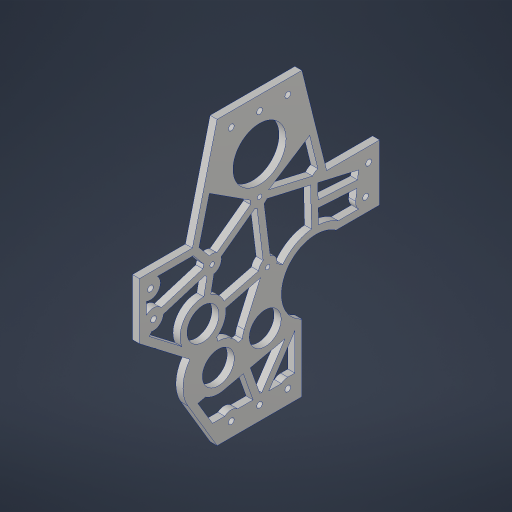
# Autodesk Inventor part: EL2-CGB-003
Saved by Autodesk Inventor 2023.4 (Build 274418000, 418)
## iProperties
Created: 2025-01-19
Part Number: EL2-CGB-003
Material: Aluminum 6061
Document SubType Name: Modeling
Designer: mavericks
Density: 2.7 g/cm^3
Appearance: Aluminum - Flat
Mass: 449.498 g
Surface Area: 622.856 cm^2
Volume: 166.481 cm^3
Author: mavericks
Autodesk Inventor part; units mm, degrees
ref_plane "YZ Plane" through (0, 0, 0) normal (1, 0, 0) x (0, 1, 0)
ref_plane "XZ Plane" through (0, 0, 0) normal (0, 1, 0) x (-1, 0, 0)
ref_plane "XY Plane" through (0, 0, 0) normal (0, 0, 1) x (1, 0, 0)
sketch "Sketch1" plane through (0, 0, 0) normal (1, 0, 0) x (0, 1, 0)
  line L0 (127, 107.95) -> (-127, 107.95) construction
  line L1 (-127, 107.95) -> (-127, 82.55) construction
  line L2 (-127, 82.55) -> (127, 82.55) construction
  line L3 (127, 82.55) -> (127, 107.95) construction
  line L4 (-44.45, 128.7526) -> (-69.85, 128.7526) construction
  line L5 (-69.85, 128.7526) -> (-69.85, 79.4258) construction
  line L6 (-69.85, 79.4258) -> (-44.45, 79.4258) construction
  line L7 (-44.45, 79.4258) -> (-44.45, 128.7526) construction
  line L8 (69.85, 128.7526) -> (44.45, 128.7526) construction
  line L9 (44.45, 128.7526) -> (44.45, 79.4258) construction
  line L10 (44.45, 79.4258) -> (69.85, 79.4258) construction
  line L11 (69.85, 79.4258) -> (69.85, 128.7526) construction
  line L12 (44.45, 104.0892) -> (-44.45, 104.0892) construction
  line L13 (0, 0) -> (-27.2932, 0) construction
  line L14 (127, -107.95) -> (-127, -107.95) construction
  line L15 (-127, -107.95) -> (-127, -82.55) construction
  line L16 (-127, -82.55) -> (127, -82.55) construction
  line L17 (127, -82.55) -> (127, -107.95) construction
  line L18 (-44.45, -128.7526) -> (-69.85, -128.7526) construction
  line L19 (-69.85, -128.7526) -> (-69.85, -79.4258) construction
  line L20 (-69.85, -79.4258) -> (-44.45, -79.4258) construction
  line L21 (-44.45, -79.4258) -> (-44.45, -128.7526) construction
  line L22 (69.85, -128.7526) -> (44.45, -128.7526) construction
  line L23 (44.45, -128.7526) -> (44.45, -79.4258) construction
  line L24 (44.45, -79.4258) -> (69.85, -79.4258) construction
  line L25 (69.85, -79.4258) -> (69.85, -128.7526) construction
  line L26 (44.45, -104.0892) -> (-44.45, -104.0892) construction
  line L27 (127, 82.55) -> (101.6, 82.55) construction
  line L28 (101.6, 82.55) -> (101.6, -82.55) construction
  line L29 (101.6, -82.55) -> (127, -82.55) construction
  line L30 (127, -82.55) -> (127, 82.55) construction
  line L31 (-127, 82.55) -> (-101.6, 82.55) construction
  line L32 (-101.6, 82.55) -> (-101.6, -82.55) construction
  line L33 (-101.6, -82.55) -> (-127, -82.55) construction
  line L34 (-127, -82.55) -> (-127, 82.55) construction
  point P0 (0, 82.55)
  point P1 (0, 104.0892)
  point P2 (0, -82.55)
  point P3 (0, -104.0892)
  dimension "d0" = 254
  dimension "d1" = 25.4
  dimension "d2" = 82.55
  dimension "d3" = 25.4
  dimension "d4" = 49.3268
  dimension "d6" = 88.9
  dimension "d7" = 3.1242
  dimension "d8" = 25.4
  dimension "d9" = 25.4
  constraints: 70 end point, 16 symmetric about line, 12 parallel, 7 horizontal, 5 perpendicular, 4 midpoint, 2 vertical alignment, 1 horizontal alignment, 1 point on line
  measures "d0" distance of L2.end L1.end
  measures "d1" distance of L1.end L0.end
  measures "d2" vertical distance of L13.start L2.end
  measures "d3" distance of L6.end L5.end
  measures "d4" distance of L5.end L4.end
  measures "d6" distance of L4.start L8.end
  measures "d7" distance from line of L2 L6.end
  measures "d8" distance between parallel lines of L28 L30
  measures "d9" distance between parallel lines of L34 L32
sketch "Sketch2" plane through (0, 0, 0) normal (1, 0, 0) x (0, 1, 0)
  line L0 (-127, 107.95) -> (-127, 82.55) construction
  line L1 (44.45, 104.0892) -> (-44.45, 104.0892) construction
  line L2 (-127, 82.55) -> (127, 82.55) construction
  line L3 (127, 107.95) -> (-127, 107.95) construction
  line L4 (44.45, 79.4258) -> (69.85, 79.4258) construction
  line L5 (127, 82.55) -> (127, 107.95) construction
  line L6 (-69.85, 79.4258) -> (-44.45, 79.4258) construction
  line L7 (-44.45, 79.4258) -> (-44.45, 128.7526) construction
  line L8 (-69.85, 128.7526) -> (-69.85, 79.4258) construction
  line L9 (-44.45, 128.7526) -> (-69.85, 128.7526) construction
  line L10 (101.6, 82.55) -> (101.6, -82.55) construction
  line L11 (127, -82.55) -> (127, 82.55) construction
  line L12 (-127, -82.55) -> (127, -82.55) construction
  line L13 (127, -107.95) -> (-127, -107.95) construction
  line L14 (44.45, -104.0892) -> (-44.45, -104.0892) construction
  line L15 (-127, 82.55) -> (-101.6, 82.55) construction
  line L16 (-101.6, 82.55) -> (-101.6, -82.55) construction
  line L17 (-127, -82.55) -> (-127, 82.55) construction
  line L18 (-69.85, -79.4258) -> (-44.45, -79.4258) construction
  line L19 (-101.6, -82.55) -> (-127, -82.55) construction
  line L20 (-44.45, -79.4258) -> (-44.45, -128.7526) construction
  line L21 (-44.45, -128.7526) -> (-69.85, -128.7526) construction
  line L22 (-69.85, -128.7526) -> (-69.85, -79.4258) construction
  line L23 (-127, -107.95) -> (-127, -82.55) construction
  line L24 (44.45, -79.4258) -> (69.85, -79.4258) construction
  line L25 (44.45, -128.7526) -> (44.45, -79.4258) construction
  line L26 (101.6, -82.55) -> (127, -82.55) construction
  line L27 (69.85, -128.7526) -> (44.45, -128.7526) construction
  line L28 (69.85, -79.4258) -> (69.85, -128.7526) construction
  line L29 (127, -82.55) -> (127, -107.95) construction
  line L30 (69.85, 128.7526) -> (44.45, 128.7526) construction
  line L31 (44.45, 128.7526) -> (44.45, 79.4258) construction
  line L32 (69.85, 79.4258) -> (69.85, 128.7526) construction
  line L33 (127, 82.55) -> (101.6, 82.55) construction
  circle A0 centre (-38.1, -50.8) radius 7.62 construction
  circle A1 centre (-57.15, -5.08) radius 41.91 construction
  circle A2 centre (-57.15, -5.08) radius 11.43 construction
  circle A3 centre (-66.675, 37.0363) radius 31.75 construction
  circle A4 centre (-66.675, 37.0363) radius 15.24 construction
  circle A5 centre (-25.7473, 50.8) radius 27.94 construction
  circle A6 centre (-38.1, -50.8) radius 31.115 construction
  circle A7 centre (-38.1, -50.8) radius 10.16 construction
  circle A8 centre (-57.15, -5.08) radius 14.2875
  circle A9 centre (-66.675, 37.0363) radius 14.2875
  circle A10 centre (-25.7473, 50.8) radius 14.2875
  circle A11 centre (-25.7473, 50.8) radius 20.6375 construction
  circle A12 centre (-66.675, 37.0363) radius 20.6375 construction
  circle A13 centre (-57.15, -5.08) radius 20.6375 construction
  circle A14 centre (-38.1, -50.8) radius 17.4625 construction
  circle A15 centre (-38.1, -50.8) radius 25.4 construction
  line L34 (-41.275, -131.9276) -> (-41.275, -76.2508) construction
  line L35 (-41.275, -76.2508) -> (-73.025, -76.2508) construction
  line L36 (-73.025, -76.2508) -> (-73.025, -131.9276) construction
  line L37 (-73.025, -131.9276) -> (-41.275, -131.9276) construction
  line L38 (-127, -38.1) -> (-127, 38.1)
  line L39 (-127, 38.1) -> (-41.275, 38.1) construction
  line L40 (-41.275, 38.1) -> (-41.275, 104.0892) construction
  circle A16 centre (-38.1, -50.8) radius 31.115
  circle A17 centre (80.9686, 0) radius 23.8125
  circle A18 centre (80.9686, 0) radius 33.3375 construction
  line L41 (37.9487, 60.325) -> (127, 38.1)
  line L42 (127, 38.1) -> (127, -38.1)
  line L43 (127, -38.1) -> (37.9487, -60.325)
  line L44 (37.9487, -60.325) -> (37.9487, -107.95)
  line L45 (37.9487, -107.95) -> (-12.7, -107.95)
  line L46 (37.9487, 60.325) -> (37.9487, 107.95)
  line L47 (37.9487, 107.95) -> (-12.7, 107.95)
  arc A19 (-23.3654, 68.8297) -> (-38.2397, 37.5831) centre (-25.7473, 50.8) ccw construction
  arc A20 (43.4827, -39.6598) -> (88.1161, 54.1018) centre (80.9686, 0) ccw construction
  line L48 (-12.7, 107.95) -> (-47.625, 62.4363)
  line L49 (-82.9044, 64.325) -> (-127, 38.1)
  arc A21 (-47.625, 62.4363) -> (-82.9044, 64.325) centre (-66.675, 37.0363) ccw
  line L50 (-66.5052, -38.1) -> (-127, -38.1)
  line L51 (-12.7, -68.7717) -> (-12.7, -107.95)
  line L52 (-23.3654, 68.8297) -> (88.1161, 54.1018) construction
  line L53 (-38.2397, 37.5831) -> (43.4827, -39.6598) construction
  point P0 (25.2487, 98.0186)
  point P1 (0, 95.25)
  point P2 (25.2487, -98.0186)
  point P3 (0, -95.25)
  point P4 (-25.4, -95.25)
  point P5 (-25.4, 95.25)
  point P6 (127, -95.25)
  point P7 (127, 95.25)
  point P8 (0, -82.55)
  point P9 (-114.3, 25.4)
  point P10 (-114.3, 0)
  point P11 (-114.3, -25.4)
  point P12 (-101.6, 0)
  point P13 (-114.3, 82.55)
  point P14 (-38.1, -25.4)
  point P15 (-38.1, -33.3375)
  point P16 (-60.097, -38.1)
  point P17 (-53.223, -42.0688)
  point P18 (-60.097, -63.5)
  point P19 (-53.223, -59.5312)
  point P20 (-38.1, -76.2)
  point P21 (-38.1, -68.2625)
  point P22 (-16.103, -63.5)
  point P23 (-22.977, -59.5313)
  point P24 (-16.103, -38.1)
  point P25 (-22.977, -42.0688)
  point P26 (44.45, 104.0892)
  point P27 (-41.275, -81.7526)
  point P28 (-127, 0)
  point P29 (-127, 0)
  point P30 (101.6, 0)
  point P31 (114.3, 25.4)
  point P32 (114.3, 0)
  point P33 (114.3, -25.4)
  point P34 (114.3, 82.55)
  point P35 (127, 0)
  dimension "d13" = 63.5
  dimension "d33" = 34.925
  dimension "d34" = 50.8
  dimension "d10" = 15.24
  dimension "d11" = 83.82
  dimension "d12" = 22.86
  dimension "d14" = 30.48
  dimension "d15" = 55.88
  dimension "d16" = 62.23
  dimension "d19" = 63.5
  dimension "d23" = 20.32
  dimension "d24" = 28.575
  dimension "d26" = 25.4
  dimension "d27" = 25.4
  dimension "d28" = 25.4
  dimension "d29" = 25.4
  dimension "d30" = 6.35
  dimension "d31" = 6.35
  dimension "d32" = 6.35
  dimension "d37" = 360
  dimension "d41" = 3.175
  dimension "d42" = 76.2
  dimension "d60" = 101.7513
  dimension "d63" = 31.75
  dimension "d64" = 44.45
  dimension "d66" = 34.925
  dimension "d67" = 31.75
  dimension "d68" = 47.625
  dimension "d70" = 9.525
  dimension "d71" = 47.625
  dimension "d73" = 118.1903
  dimension "d74" = 12.7
  dimension "d75" = 36.3728
  dimension "d76" = 109.1438
  dimension "d78" = 9.9314
  dimension "d79" = 9.9314
  dimension "d137" = 12.7
  dimension "d149" = 205.5979
  dimension "d151" = 45.7518
  dimension "d152" = 112.4501
  dimension "d153" = 6.35
  constraints: 41 end point, 19 centre point, 18 vertical alignment, 14 coincident, 11 horizontal alignment, 11 midpoint, 10 point on circle, 9 point on line, 6 tangent, 3 perpendicular, 2 collinear, 2 equal radius, 2 horizontal, 1 vertical, 25 other
  measures "d10" diameter of A0
  measures "d11" diameter of A1
  measures "d12" diameter of A2
  measures "d14" diameter of A4
  measures "d15" diameter of A5
  measures "d16" diameter of A6
  measures "d19" distance from line of L16 A0.centre
  measures "d23" diameter of A7
  measures "d24" diameter of A8
  measures "d26" distance of point (-25.4, 95.25) point (0, 95.25)
  measures "d27" distance of point (25.249, 98.019) point (0, 95.25)
  measures "d28" distance of point (-114.3, 0) point (-114.3, 25.4)
  measures "d29" distance of point (-114.3, 0) point (-114.3, -25.4)
  measures "d30" radial gap between concentric circles of A10 A11
  measures "d31" radial gap between concentric circles of A9 A12
  measures "d32" radial gap between concentric circles of A8 A13
  measures "d41" distance between parallel lines of L20 L34
  measures "d42" distance of L38.start L38.end
  measures "d60" distance from line of L5 point (25.249, 98.019)
  measures "d63" distance from line of L12 A0.centre
  measures "d64" distance from line of L16 A1.centre
  measures "d66" distance from line of L16 point (-66.675, 37.036)
  measures "d67" distance from line of L2 A5.centre
  measures "d68" diameter of A17
  measures "d70" radial gap between concentric circles of A17 A18
  measures "d71" distance of L41.start L46.end
  measures "d73" distance of A17.centre A5.centre
  measures "d74" horizontal distance of point (25.249, 98.019) L46.end
  measures "d75" diameter of A19
  measures "d76" diameter of A20
  measures "d78" distance from line of point (25.249, 98.019) L3
  measures "d79" distance from line of L13 point (25.249, -98.019)
  measures "d137" distance from line of L51 point (0, -95.25)
  measures "d152" distance of L52.start L52.end
  measures "d153" distance from line of L40 L48.end
extrude "Extrusion1" add sketch "Sketch2" along normal blind 6.35 contours L38 L49 A21 L48 L47 L46 L41 L42 L43 L44 L45 L51 A16 L50
hole "Mount Holes" at (0, -101.6, 82.55) at (0, -127, 107.95) at (0, -69.85, 79.4258) at (0, -44.45, -79.4258) at (0, 44.45, -79.4258) at (0, 69.85, -79.4258) at (0, 44.45, -128.7526) at (0, 44.45, 128.7526) at (0, 25.2487, 98.0186) at (0, 0, 95.25) at (0, 25.2487, -98.0186) at (0, 0, -95.25) at (0, -25.4, -95.25) at (0, -25.4, 95.25) at (0, -114.3, 25.4) at (0, -114.3, 0) at (0, -114.3, -25.4) at (0, 114.3, 25.4) at (0, 114.3, 0) at (0, 114.3, -25.4) direction (1, 0, 0) diameter 5.1054 end through all clearance for "Flat Head Machine Screw (82)" size "#10" standard "Ansi Unified Screw Threads"
sketch "Sketch7" plane through (6.35, 0, 0) normal (1, 0, 0) x (0, 0, -1)
  circle A0 centre (0, 114.3) radius 2.5527 construction
  circle A1 centre (25.4, -114.3) radius 2.5527 construction
  circle A2 centre (-25.4, -114.3) radius 2.5527 construction
  circle A3 centre (98.0186, 25.2487) radius 2.5527 construction
  circle A4 centre (-98.0186, 25.2487) radius 2.5527 construction
  circle A5 centre (-95.25, 0) radius 2.5527 construction
  circle A6 centre (95.25, 0) radius 2.5527 construction
  circle A7 centre (0, -114.3) radius 2.5527 construction
  circle A8 centre (-25.4, 114.3) radius 2.5527 construction
  circle A9 centre (25.4, 114.3) radius 2.5527 construction
  circle A10 centre (5.08, -57.15) radius 14.2875 construction
  circle A11 centre (-37.0363, -66.675) radius 14.2875 construction
  circle A12 centre (-50.8, -25.7473) radius 14.2875 construction
  circle A13 centre (0, 80.9686) radius 23.8125 construction
  line L0 (38.1, -127) -> (-38.1, -127) construction
  line L1 (-38.1, -127) -> (-64.325, -82.9044) construction
  arc A14 (-62.4363, -47.625) -> (-64.325, -82.9044) centre (-37.0363, -66.675) ccw construction
  line L2 (-62.4363, -47.625) -> (-93.0211, -24.1557) construction
  arc A15 (-93.0211, -24.1557) -> (-94.6249, -22.925) centre (-95.25, -25.4) ccw construction
  line L3 (-94.6249, -22.925) -> (-107.95, -12.7) construction
  line L4 (-107.95, -12.7) -> (-107.95, 37.9487) construction
  line L5 (-107.95, 37.9487) -> (-60.325, 37.9487) construction
  line L6 (-60.325, 37.9487) -> (-38.1, 127) construction
  line L7 (-38.1, 127) -> (38.1, 127) construction
  line L8 (38.1, 127) -> (60.325, 37.9487) construction
  line L9 (60.325, 37.9487) -> (107.95, 37.9487) construction
  line L10 (107.95, 37.9487) -> (107.95, -12.7) construction
  line L11 (107.95, -12.7) -> (68.7717, -12.7) construction
  arc A16 (68.7717, -12.7) -> (38.1, -66.5052) centre (50.8, -38.1) ccw construction
  line L12 (38.1, -66.5052) -> (38.1, -127) construction
  circle A17 centre (0, 80.9686) radius 54.5719 construction
  circle A18 centre (-50.8, -25.7473) radius 18.1864 construction
  line L13 (-54.1018, 88.1161) -> (-68.8297, -23.3654) construction
  line L14 (-37.5831, -38.2397) -> (39.6598, 43.4827) construction
  circle A19 centre (5.08, -2.5527) radius 20.6375 construction
  line L15 (-4.4521, -30.1851) -> (53.1372, 30.744) construction
  circle A20 centre (-4.4521, -30.1851) radius 4.7625 construction
  circle A21 centre (53.1372, 30.744) radius 4.7625 construction
  point P0 (0, 0)
  dimension "d154" = 109.1438
  dimension "d155" = 36.3728
  dimension "d194" = 41.275
  dimension "d197" = 9.525
  dimension "d198" = 9.525
  constraints: 6 end point, 5 centre point, 4 coincident, 4 point on circle, 4 tangent, 1 parallel
  measures "d154" diameter of A17
  measures "d155" diameter of A18
  measures "d194" diameter of A19
  measures "d197" diameter of A20
  measures "d198" diameter of A21
hole "Hole4" [suppressed]
sketch "Sketch8" plane through (6.35, 0, 0) normal (1, 0, 0) x (0, 0, -1)
  circle A0 centre (0, 114.3) radius 2.5527 construction
  line L0 (0, 47.6504) -> (0, 114.3) construction
  point P0 (0, 0)
  dimension "d183" = 66.6496
  constraints: 2 end point, 1 vertical
  measures "d183" distance of L0.start L0.end
hole "Hole5" at (6.35, 47.6504, 0) direction (-1, 0, 0) diameter 3.9624 end through all thread size "10-32 UNF" class "2B" standard "ANSI Unified Screw Threads"
sketch "Sketch9" plane through (0, 0, 0) normal (-1, 0, 0) x (0, 0, 1)
  circle A0 centre (0, 47.6504) radius 1.9812 construction
  circle A1 centre (0, 114.3) radius 2.5527 construction
  circle A2 centre (-25.4, -114.3) radius 2.5527 construction
  circle A3 centre (25.4, -114.3) radius 2.5527 construction
  circle A4 centre (-98.0186, 25.2487) radius 2.5527 construction
  circle A5 centre (98.0186, 25.2487) radius 2.5527 construction
  circle A6 centre (95.25, 0) radius 2.5527 construction
  circle A7 centre (-95.25, 0) radius 2.5527 construction
  circle A8 centre (0, -114.3) radius 2.5527 construction
  circle A9 centre (25.4, 114.3) radius 2.5527 construction
  circle A10 centre (-25.4, 114.3) radius 2.5527 construction
  circle A11 centre (-5.08, -57.15) radius 14.2875 construction
  circle A12 centre (37.0363, -66.675) radius 14.2875 construction
  circle A13 centre (50.8, -25.7473) radius 14.2875 construction
  circle A14 centre (0, 80.9686) radius 23.8125 construction
  line L0 (38.1, -127) -> (-38.1, -127) construction
  line L1 (-38.1, -127) -> (-38.1, -66.5052) construction
  arc A15 (-38.1, -66.5052) -> (-68.7717, -12.7) centre (-50.8, -38.1) ccw construction
  line L2 (-68.7717, -12.7) -> (-107.95, -12.7) construction
  line L3 (-107.95, -12.7) -> (-107.95, 37.9487) construction
  line L4 (-107.95, 37.9487) -> (-60.325, 37.9487) construction
  line L5 (-60.325, 37.9487) -> (-38.1, 127) construction
  line L6 (-38.1, 127) -> (38.1, 127) construction
  line L7 (38.1, 127) -> (60.325, 37.9487) construction
  line L8 (60.325, 37.9487) -> (107.95, 37.9487) construction
  line L9 (107.95, 37.9487) -> (107.95, -12.7) construction
  line L10 (107.95, -12.7) -> (94.6249, -22.925) construction
  arc A16 (94.6249, -22.925) -> (93.0211, -24.1557) centre (95.25, -25.4) ccw construction
  line L11 (93.0211, -24.1557) -> (62.4363, -47.625) construction
  arc A17 (64.325, -82.9044) -> (62.4363, -47.625) centre (37.0363, -66.675) ccw construction
  line L12 (64.325, -82.9044) -> (38.1, -127) construction
  circle A18 centre (50.8, -25.7473) radius 14.2875 construction
  circle A19 centre (50.8, -25.7473) radius 18.1864 construction
  circle A20 centre (0, 80.9686) radius 54.5719 construction
  line L13 (54.1018, 88.1161) -> (68.8297, -23.3654) construction
  line L14 (-39.6598, 43.4827) -> (37.5831, -38.2397) construction
  circle A21 centre (17.6097, 2.7489) radius 13.6398 construction
  line L15 (-7.4011, -10.7665) -> (42.6205, 16.2642) construction
  line L16 (0, 80.9686) -> (50.8, -25.7473) construction
  line L17 (23.4558, 31.6947) -> (42.9832, -9.3265) construction
  point P0 (0, 0)
  point P1 (33.2195, 11.1841)
  dimension "d199" = 28.575
  dimension "d201" = 36.3728
  dimension "d202" = 109.1438
  dimension "d204" = 50.8
  dimension "d205" = 106.716
  dimension "d206" = 27.2796
  dimension "d207" = 56.8579
  dimension "d208" = 75
  constraints: 10 end point, 6 point on circle, 5 coincident, 5 tangent, 3 centre point, 3 point on line, 2 midpoint
  measures "d199" diameter of A13
  measures "d201" diameter of A19
  measures "d202" diameter of A20
  measures "d204" horizontal distance of A13.centre L16.start
  measures "d205" vertical distance of A13.centre A14.centre
  measures "d206" diameter of A21
  measures "d207" distance of L15.start L15.end
  measures "d208" angle of L14 L15
hole "Hole6" at (0, 16.2642, 42.6205) at (0, -10.7665, -7.4011) at (0, 16.2642, 42.6205) direction (1, 0, 0) diameter 3.9624 end through all thread size "10-32 UNF" class "2B" standard "ANSI Unified Screw Threads"
sketch "Sketch10" plane through (6.35, 0, 0) normal (1, 0, 0) x (0, 0, -1)
  circle A0 centre (7.4011, -10.7665) radius 1.9812 construction
  circle A1 centre (-42.6205, 16.2642) radius 1.9812 construction
  circle A2 centre (0, 47.6504) radius 1.9812 construction
  circle A3 centre (0, 114.3) radius 2.5527 construction
  circle A4 centre (25.4, -114.3) radius 2.5527 construction
  circle A5 centre (-25.4, -114.3) radius 2.5527 construction
  circle A6 centre (98.0186, 25.2487) radius 2.5527 construction
  circle A7 centre (-98.0186, 25.2487) radius 2.5527 construction
  circle A8 centre (-95.25, 0) radius 2.5527 construction
  circle A9 centre (95.25, 0) radius 2.5527 construction
  circle A10 centre (0, -114.3) radius 2.5527 construction
  circle A11 centre (-25.4, 114.3) radius 2.5527 construction
  circle A12 centre (25.4, 114.3) radius 2.5527 construction
  circle A13 centre (5.08, -57.15) radius 14.2875 construction
  circle A14 centre (-37.0363, -66.675) radius 14.2875 construction
  circle A15 centre (-50.8, -25.7473) radius 14.2875 construction
  circle A16 centre (0, 80.9686) radius 23.8125 construction
  line L0 (38.1, -127) -> (-38.1, -127) construction
  line L1 (-38.1, -127) -> (-64.325, -82.9044) construction
  arc A17 (-62.4363, -47.625) -> (-64.325, -82.9044) centre (-37.0363, -66.675) ccw construction
  line L2 (-62.4363, -47.625) -> (-93.0211, -24.1557) construction
  arc A18 (-93.0211, -24.1557) -> (-94.6249, -22.925) centre (-95.25, -25.4) ccw construction
  line L3 (-94.6249, -22.925) -> (-107.95, -12.7) construction
  line L4 (-107.95, -12.7) -> (-107.95, 37.9487) construction
  line L5 (-107.95, 37.9487) -> (-60.325, 37.9487) construction
  line L6 (-60.325, 37.9487) -> (-38.1, 127) construction
  line L7 (-38.1, 127) -> (38.1, 127) construction
  line L8 (38.1, 127) -> (60.325, 37.9487) construction
  line L9 (60.325, 37.9487) -> (107.95, 37.9487) construction
  line L10 (107.95, 37.9487) -> (107.95, -12.7) construction
  line L11 (107.95, -12.7) -> (68.7717, -12.7) construction
  arc A19 (68.7717, -12.7) -> (38.1, -66.5052) centre (50.8, -38.1) ccw construction
  line L12 (38.1, -66.5052) -> (38.1, -127) construction
  line L13 (-33.14, 120.65) -> (-55.365, 31.5987) construction
  line L14 (-55.365, 31.5987) -> (-101.6, 31.5987) construction
  line L15 (-101.6, 31.5987) -> (-101.6, -9.5686) construction
  line L16 (-101.6, -9.5686) -> (-91.4775, -17.3361) construction
  arc A20 (-88.4371, -19.6692) -> (-91.4775, -17.3361) centre (-95.25, -25.4) ccw construction
  line L17 (-88.4371, -19.6692) -> (-52.9641, -46.8895) construction
  arc A21 (-52.9641, -46.8895) -> (-58.8673, -79.6585) centre (-37.0363, -66.675) ccw construction
  line L18 (-58.8673, -79.6585) -> (-34.4884, -120.65) construction
  line L19 (-34.4884, -120.65) -> (31.75, -120.65) construction
  line L20 (31.75, -120.65) -> (31.75, -70.3602) construction
  arc A22 (70.6888, -6.35) -> (31.75, -70.3602) centre (50.8, -38.1) ccw construction
  line L21 (70.6888, -6.35) -> (101.6, -6.35) construction
  line L22 (101.6, -6.35) -> (101.6, 31.5987) construction
  line L23 (101.6, 31.5987) -> (55.365, 31.5987) construction
  line L24 (55.365, 31.5987) -> (33.14, 120.65) construction
  line L25 (33.14, 120.65) -> (-33.14, 120.65) construction
  circle A23 centre (0, 47.6504) radius 1.9812 construction
  circle A24 centre (0, 47.6504) radius 8.3312 construction
  circle A25 centre (98.0186, 25.2487) radius 8.9027 construction
  circle A26 centre (95.25, 0) radius 8.9027 construction
  circle A27 centre (7.4011, -10.7665) radius 8.3312 construction
  circle A28 centre (-42.6205, 16.2642) radius 8.3312 construction
  circle A29 centre (-50.8, -25.7473) radius 20.6375 construction
  circle A30 centre (-98.0186, 25.2487) radius 8.9027 construction
  circle A31 centre (-95.25, 0) radius 8.9027 construction
  circle A32 centre (5.08, -57.15) radius 20.6375 construction
  circle A33 centre (-37.0363, -66.675) radius 20.6375 construction
  circle A34 centre (25.4, -114.3) radius 8.9027 construction
  circle A35 centre (0, -114.3) radius 8.9027 construction
  circle A36 centre (-25.4, -114.3) radius 8.9027 construction
  line L26 (-32.484, -86.8041) -> (9.6324, -77.2791) construction
  circle A37 centre (0, -114.3) radius 2.5527 construction
  line L27 (0, -114.3) -> (-11.4258, -82.0416) construction
  circle A38 centre (7.4011, -10.7665) radius 1.9812 construction
  line L28 (-50.8, -25.7473) -> (7.4011, -10.7665) construction
  line L29 (7.4011, -10.7665) -> (50.8, -38.1) construction
  line L30 (-36.518, -25.3497) -> (6.8672, -14.1824) construction
  line L31 (6.8672, -14.1824) -> (75.2988, -57.2821) construction
  line L32 (-38.1009, -19.2001) -> (7.9351, -7.3505) construction
  line L33 (7.9351, -7.3505) -> (78.6829, -51.909) construction
  arc A39 (68.7717, -12.7) -> (38.1, -66.5052) centre (50.8, -38.1) ccw construction
  circle A40 centre (-50.8, -25.7473) radius 14.2875 construction
  line L34 (7.4011, -10.7665) -> (0, 47.6504) construction
  line L35 (0, 47.6504) -> (98.0186, 25.2487) construction
  line L36 (0, 47.6504) -> (-42.6205, 16.2642) construction
  line L37 (-42.6205, 16.2642) -> (-50.8, -25.7473) construction
  circle A41 centre (-42.6205, 16.2642) radius 1.9812 construction
  line L38 (-42.6205, 16.2642) -> (-55.365, 31.5987) construction
  circle A42 centre (-95.25, 0) radius 2.5527 construction
  line L39 (-95.25, 0) -> (-42.6205, 16.2642) construction
  line L40 (49.0093, 36.4495) -> (50.8, -38.1) construction
  line L41 (45.8945, 33.9045) -> (46.8826, -7.2326) construction
  line L42 (52.2814, 32.4448) -> (54.7174, -68.9674) construction
  line L43 (105.4194, 20.3004) -> (0.7111, 44.231) construction
  line L44 (0.7111, 44.231) -> (-39.7407, 14.4419) construction
  line L45 (-39.7407, 14.4419) -> (-50.3457, -40.0276) construction
  line L46 (-104.1339, 0.5777) -> (-48.1027, 17.8932) construction
  line L47 (-48.1027, 17.8932) -> (-59.4934, 31.5987) construction
  line L48 (-2.1817, 39.6099) -> (3.2832, -3.5241) construction
  line L49 (4.118, 40.4081) -> (9.5828, -2.726) construction
  line L50 (-13.8121, -48.8437) -> (0.7332, -15.7613) construction
  line L51 (-38.5221, -42.3353) -> (-37.2767, -46.0389) construction
  line L52 (-19.2845, -56.1499) -> (-15.4733, -55.288) construction
  line L53 (-37.0363, -66.675) -> (5.08, -57.15) construction
  line L54 (-50.8, -25.7473) -> (-37.0363, -66.675) construction
  line L55 (-5.7697, -107.52) -> (-14.5443, -82.7469) construction
  line L56 (5.7697, -121.08) -> (-8.3073, -81.3364) construction
  line L57 (-42.2972, -107.52) -> (31.75, -107.52) construction
  line L58 (-48.4099, -83.8956) -> (-55.4063, -85.4779) construction
  line L59 (45.8945, 33.9045) -> (46.7295, -0.8568)
  line L60 (4.118, 40.4081) -> (9.5828, -2.726)
  arc A43 (15.6107, -12.1848) -> (9.5828, -2.726) centre (7.4011, -10.7665) ccw
  line L61 (15.6107, -12.1848) -> (20.9047, -15.5191)
  arc A44 (46.7295, -0.8568) -> (20.9047, -15.5191) centre (50.8, -38.1) ccw
  line L62 (45.8945, 33.9045) -> (6.8015, 42.8391)
  arc A45 (4.118, 40.4081) -> (6.8015, 42.8391) centre (0, 47.6504) ccw
  line L63 (-4.3195, 40.5264) -> (-34.5356, 18.275)
  line L64 (-40.976, 8.0969) -> (-43.7865, -6.3381)
  line L65 (-31.8433, -17.5894) -> (-0.8496, -9.6117)
  line L66 (3.2832, -3.5241) -> (-2.1817, 39.6099)
  arc A46 (-4.3195, 40.5264) -> (-2.1817, 39.6099) centre (0, 47.6504) ccw
  arc A47 (-40.976, 8.0969) -> (-34.5356, 18.275) centre (-42.6205, 16.2642) ccw
  arc A48 (-31.8433, -17.5894) -> (-43.7865, -6.3381) centre (-50.8, -25.7473) ccw
  arc A49 (3.2832, -3.5241) -> (-0.8496, -9.6117) centre (7.4011, -10.7665) ccw
  line L67 (-86.3661, -0.5777) -> (-49.0421, 10.9565) construction
  line L68 (-50.0194, -5.1246) -> (-47.209, 9.3104) construction
  line L69 (-86.3661, -0.5777) -> (-49.0421, 10.9565)
  line L70 (-47.209, 9.3104) -> (-50.0194, -5.1246)
  line L71 (-99.0811, -11.5014) -> (-69.6924, -34.0529)
  line L72 (-96.9598, -8.737) -> (-99.0811, -11.5014) construction
  circle A50 centre (0, 80.9686) radius 30.1625 construction
  circle A51 centre (0, 47.6504) radius 1.9812 construction
  line L73 (0, 47.6504) -> (-44.2525, 76.1243) construction
  line L74 (0, 47.6504) -> (44.2525, 76.1243) construction
  line L75 (45.0644, 72.8713) -> (0, 43.8749) construction
  line L76 (0, 43.8749) -> (-45.0644, 72.8713) construction
  line L77 (-99.0811, -11.5014) -> (-96.9598, -8.737)
  arc A52 (-50.0194, -5.1246) -> (-69.6924, -34.0529) centre (-50.8, -25.7473) ccw
  arc A53 (-49.0421, 10.9565) -> (-47.209, 9.3104) centre (-42.6205, 16.2642) ccw
  arc A54 (-96.9598, -8.737) -> (-86.3661, -0.5777) centre (-95.25, 0) ccw
  line L78 (53.0777, -0.7043) -> (52.2814, 32.4448) construction
  line L79 (52.6795, 15.8703) -> (87.7846, 13.5947) construction
  line L80 (86.4003, 0.9704) -> (89.1689, 26.2191) construction
  line L81 (52.603, 19.0569) -> (88.1311, 16.7539) construction
  line L82 (52.7561, 12.6836) -> (87.4382, 10.4355) construction
  line L83 (87.4382, 10.4355) -> (52.7561, 12.6836)
  line L84 (52.7561, 12.6836) -> (53.0777, -0.7043)
  line L85 (87.4382, 10.4355) -> (86.4003, 0.9704)
  line L86 (89.0102, -6.35) -> (70.6888, -6.35)
  arc A55 (70.6888, -6.35) -> (53.0777, -0.7043) centre (50.8, -38.1) ccw
  circle A56 centre (95.25, 0) radius 2.5527 construction
  arc A57 (86.4003, 0.9704) -> (89.0102, -6.35) centre (95.25, 0) ccw
  line L87 (52.2814, 32.4448) -> (88.9331, 24.0682)
  line L88 (88.9331, 24.0682) -> (88.1311, 16.7539)
  line L89 (88.1311, 16.7539) -> (52.603, 19.0569)
  line L90 (52.603, 19.0569) -> (52.2814, 32.4448)
  line L91 (-38.301, 23.3881) -> (-8.0849, 45.6396) construction
  line L92 (8.2163, 49.0295) -> (53.6036, 38.6564) construction
  line L93 (-54.4116, 35.4188) -> (-45.1019, 24.2173) construction
  circle A58 centre (54.4656, 35.2025) radius 8.3312 construction
  line L94 (45.0644, 72.8713) -> (8.1955, 49.1482)
  line L95 (8.2163, 49.0295) -> (47.6641, 40.0138)
  line L96 (45.0644, 72.8713) -> (52.4482, 43.2858)
  arc A59 (52.4482, 43.2858) -> (47.6641, 40.0138) centre (54.4656, 35.2025) ccw
  arc A60 (8.2163, 49.0295) -> (8.1955, 49.1482) centre (0, 47.6504) ccw
  line L97 (-45.0644, 72.8713) -> (-54.4116, 35.4188)
  line L98 (-54.4116, 35.4188) -> (-45.1019, 24.2173)
  line L99 (-45.0644, 72.8713) -> (-8.1955, 49.1482)
  line L100 (-38.301, 23.3881) -> (-8.0849, 45.6396)
  arc A61 (-8.1955, 49.1482) -> (-8.0849, 45.6396) centre (0, 47.6504) ccw
  arc A62 (-38.301, 23.3881) -> (-45.1019, 24.2173) centre (-42.6205, 16.2642) ccw
  line L101 (-91.7788, 31.5987) -> (-59.4934, 31.5987)
  line L102 (-59.4934, 31.5987) -> (-49.9855, 20.1585)
  line L103 (-50.917, 17.0235) -> (-88.2409, 5.4892)
  line L104 (-101.6, 17.0981) -> (-101.6, 6.2398)
  arc A63 (-88.2409, 5.4892) -> (-101.6, 6.2398) centre (-95.25, 0) ccw
  arc A64 (-101.6, 17.0981) -> (-91.7788, 31.5987) centre (-98.0186, 25.2487) ccw
  arc A65 (-49.9855, 20.1585) -> (-50.917, 17.0235) centre (-42.6205, 16.2642) ccw
  line L105 (-30.2605, -23.739) -> (0.7332, -15.7613)
  line L106 (0.7332, -15.7613) -> (-13.8121, -48.8437)
  line L107 (-19.2845, -56.1499) -> (-15.4733, -55.288)
  line L108 (-38.5221, -42.3353) -> (-37.2767, -46.0389)
  circle A66 centre (-50.8, -25.7473) radius 14.2875 construction
  arc A67 (-38.5221, -42.3353) -> (-30.2605, -23.739) centre (-50.8, -25.7473) ccw
  arc A68 (-19.2845, -56.1499) -> (-37.2767, -46.0389) centre (-37.0363, -66.675) ccw
  circle A69 centre (5.08, -57.15) radius 14.2875 construction
  arc A70 (-13.8121, -48.8437) -> (-15.4733, -55.288) centre (5.08, -57.15) ccw
  line L109 (0, -114.3) -> (50.8, -38.1) construction
  line L110 (7.2554, -109.1408) -> (31.75, -72.3988) construction
  line L111 (1.9718, -105.6184) -> (27.4512, -67.3995) construction
  line L112 (-14.5443, -82.7469) -> (-5.7697, -107.52)
  line L113 (-5.7697, -107.52) -> (-19.6303, -107.52)
  line L114 (-14.5443, -82.7469) -> (-32.484, -86.8041)
  line L115 (-55.4063, -85.4779) -> (-48.4099, -83.8956)
  line L116 (-55.4063, -85.4779) -> (-42.2972, -107.52)
  line L117 (-42.2972, -107.52) -> (-31.1697, -107.52)
  arc A71 (-48.4099, -83.8956) -> (-32.484, -86.8041) centre (-37.0363, -66.675) ccw
  arc A72 (-19.6303, -107.52) -> (-31.1697, -107.52) centre (-25.4, -114.3) ccw
  line L118 (9.6324, -77.2791) -> (27.3522, -73.2716) construction
  line L119 (-8.3073, -81.3364) -> (22.8589, -74.2878)
  line L120 (22.8589, -74.2878) -> (1.9718, -105.6184)
  arc A73 (1.9718, -105.6184) -> (0.2159, -105.3999) centre (0, -114.3) ccw
  line L121 (-8.3073, -81.3364) -> (0.2159, -105.3999)
  line L122 (31.75, -72.3988) -> (8.3359, -107.52)
  line L123 (31.75, -72.3988) -> (31.75, -105.3973)
  line L124 (25.4, -105.3973) -> (31.75, -105.3973) construction
  line L125 (31.75, -105.3973) -> (25.4, -105.3973)
  circle A74 centre (25.4, -114.3) radius 2.5527 construction
  arc A75 (25.4, -105.3973) -> (19.6303, -107.52) centre (25.4, -114.3) ccw
  line L126 (19.6303, -107.52) -> (8.3359, -107.52)
  point P0 (0, 0)
  dimension "d258" = 16.6624
  dimension "d216" = 6.35
  dimension "d218" = 6.35
  dimension "d219" = 6.35
  dimension "d220" = 6.35
  dimension "d221" = 6.35
  dimension "d222" = 6.35
  dimension "d223" = 6.35
  dimension "d224" = 6.35
  dimension "d225" = 6.35
  dimension "d226" = 6.35
  dimension "d227" = 6.35
  dimension "d228" = 6.35
  dimension "d229" = 6.35
  dimension "d230" = 6.35
  dimension "d231" = 3.175
  dimension "d232" = 3.175
  dimension "d233" = 3.175
  dimension "d234" = 3.175
  dimension "d235" = 3.175
  dimension "d236" = 3.175
  dimension "d237" = 3.175
  dimension "d238" = 3.175
  dimension "d239" = 6.35
  dimension "d240" = 6.35
  dimension "d241" = 3.175
  dimension "d242" = 3.175
  dimension "d243" = 6.35
  dimension "d246" = 3.175
  dimension "d247" = 3.175
  dimension "d248" = 3.175
  dimension "d249" = 6.35
  dimension "d250" = 3.175
  dimension "d251" = 3.175
  dimension "d252" = 3.175
  dimension "d253" = 3.175
  dimension "d254" = 3.175
  dimension "d256" = 3.175
  dimension "d257" = 16.6624
  dimension "d259" = 3.175
  dimension "d260" = 3.175
  constraints: 231 end point, 110 point on line, 104 point on circle, 40 centre point, 26 coincident, 19 parallel, 10 concentric, 6 midpoint, 4 tangent, 2 collinear, 2 horizontal, 2 perpendicular, 1 vertical alignment, 34 other
  measures "d216" distance between parallel lines of L6 L13
  measures "d218" radial gap between concentric circles of A2 A24
  measures "d219" radial gap between concentric circles of A6 A25
  measures "d221" radial gap between concentric circles of A0 A27
  measures "d222" radial gap between concentric circles of A1 A28
  measures "d223" radial gap between concentric circles of A15 A29
  measures "d225" radial gap between concentric circles of A8 A31
  measures "d226" radial gap between concentric circles of A13 A32
  measures "d227" radial gap between concentric circles of A14 A33
  measures "d229" radial gap between concentric circles of A10 A35
  measures "d230" radial gap between concentric circles of A5 A36
  measures "d231" distance between parallel lines of L28 L30
  measures "d232" distance between parallel lines of L28 L32
  measures "d233" distance between parallel lines of L40 L41
  measures "d234" distance between parallel lines of L40 L42
  measures "d235" distance between parallel lines of L35 L43
  measures "d236" distance between parallel lines of L39 L46
  measures "d237" distance between parallel lines of L34 L48
  measures "d238" distance between parallel lines of L49 L34
  measures "d239" distance between parallel lines of L54 L51
  measures "d240" distance from line of A14.centre L52
  measures "d241" distance between parallel lines of L27 L55
  measures "d242" distance between parallel lines of L27 L56
  measures "d243" distance between parallel lines of L26 L58
  measures "d246" distance between parallel lines of L37 L68
  measures "d247" distance between parallel lines of L39 L67
  measures "d248" distance of L72.end L15.end
  measures "d249" radial gap between concentric circles of A16 A50
  measures "d250" distance between parallel lines of L74 L75
  measures "d251" distance between parallel lines of L79 L81
  measures "d252" distance between parallel lines of L79 L82
  measures "d253" distance between parallel lines of L35 L92
  measures "d254" distance between parallel lines of L36 L91
  measures "d256" distance between parallel lines of L38 L93
  measures "d257" diameter of A24
  measures "d259" distance between parallel lines of L109 L110
  measures "d260" distance between parallel lines of L111 L109
extrude "Extrusion5" cut sketch "Sketch10" against normal through all
equation "\"offset\" = 6.35"
body "Solid1"
